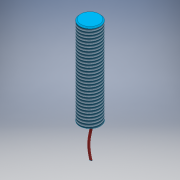
# Autodesk Inventor part: Modello sensore ultrasuoni
Saved by Autodesk Inventor 2018 (Build 220112000, 112)
## iProperties
Created: 2020-06-12
Part Number: Modello sensore ultrasuoni
Material: Plastica ABS
Document SubType Name: Modeling
Designer: Francesco
Density: 1.06 g/cm^3
Appearance: Celeste medio
Author: Francesco
Autodesk Inventor part; units mm, degrees
ref_plane "YZ Plane" through (0, 0, 0) normal (1, 0, 0) x (0, 1, 0)
ref_plane "XZ Plane" through (0, 0, 0) normal (0, 1, 0) x (-1, 0, 0)
ref_plane "XY Plane" through (0, 0, 0) normal (0, 0, 1) x (1, 0, 0)
sketch "Schizzo1" plane through (0, 0, 0) normal (0, 0, 1) x (1, 0, 0)
  circle A0 centre (0, 0) radius 9
  dimension "d0" = 18
  constraints: 1 centre point, 1 coincident
  measures "d0" diameter of A0
extrude "Estrusione1" add sketch "Schizzo1" along normal blind 77
thread "Filettatura1"
chamfer "Smusso1" distance 1 angle 45 1 edges at (-9, 0, 77)
sketch "Schizzo3" plane through (0, 0, 0) normal (0, 0, -1) x (-1, 0, 0)
  circle A0 centre (0, 0) radius 1
  dimension "d8" = 2
  constraints: 2 coincident, 1 centre point
  measures "d8" diameter of A0
sketch "Schizzo4" plane through (0, 0, 0) normal (1, 0, 0) x (0, 1, 0)
  line L0 (-9, 0) -> (9, 0) projected
  line L1 (3.6716, 0) -> (6.4362, -4.8477) construction
  line L2 (6.4362, -4.8477) -> (2.6524, -12.3111) construction
  line L3 (2.6524, -12.3111) -> (0, -13.9912) construction
  line L4 (0, -13.9912) -> (4.2654, -31.599) construction
  spline S0 degree 4 poles (3.6716, 0) (6.4362, -4.8477) (2.6524, -12.3111) (0, -13.9912) (4.2654, -31.599) knots 1 1 1 1 1 2 2 2 2 2
  point P0 (0, 0)
  constraints: 1 point on line, 3 other
sweep "Sweep1" add profiles "Schizzo3" path "Schizzo4" path curves S0
